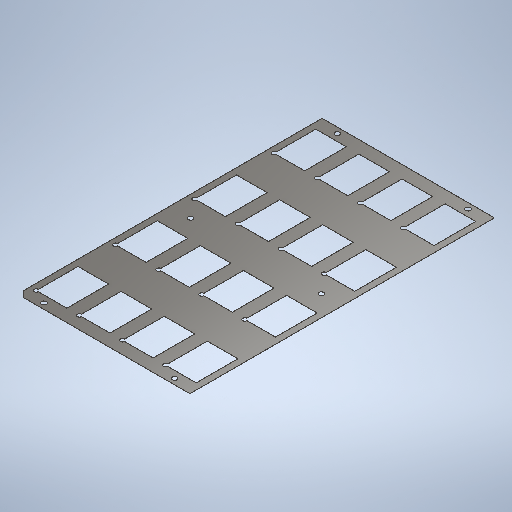
# Autodesk Inventor part: Assembly Stencil
Saved by Autodesk Inventor 2025 (Build 290162000, 162)
## iProperties
Created: 2021-01-11
Part Number: Assembly Stencil
Material: Stainless Steel
Document SubType Name: Modeling
Designer: caleb
Density: 8 g/cm^3
Appearance: Semi-Polished
Author: caleb
Autodesk Inventor part; units mm, degrees
ref_plane "YZ Plane" through (0, 0, 0) normal (1, 0, 0) x (0, 1, 0)
ref_plane "XZ Plane" through (0, 0, 0) normal (0, 1, 0) x (-1, 0, 0)
ref_plane "XY Plane" through (0, 0, 0) normal (0, 0, 1) x (1, 0, 0)
sketch "Sketch1" plane through (0, 0, 0) normal (0, 1, 0) x (-1, 0, 0)
  line L0 (-62, 109.5) -> (62, 109.5)
  line L1 (62, 109.5) -> (62, -109.5)
  line L2 (62, -109.5) -> (-62, -109.5)
  line L3 (-62, -109.5) -> (-62, 109.5)
  line L4 (-62, 109.5) -> (62, -109.5) construction
  line L5 (62, 109.5) -> (-62, -109.5) construction
  point P0 (0, 0)
  dimension "d0" = 219
  dimension "d1" = 124
  constraints: 12 end point, 2 midpoint, 2 parallel, 1 horizontal, 1 perpendicular
  measures "d0" distance of L0.end L1.end
  measures "d1" distance of L0.start L0.end
extrude "Extrusion1" add sketch "Sketch1" along normal blind 0.1
chamfer "Chamfer1" distance 4 angle 45 1 edges at (-62, 0.05, 109.5)
sketch "Sketch2" plane through (0, 0.1, 0) normal (0, 1, 0) x (1, 0, 0)
  line L0 (-35.5, -100.5) -> (-35.5, -70.5)
  line L1 (-35.5, -70.5) -> (-57.5, -70.5)
  line L2 (-62, 109.5) -> (-62, -109.5) projected
  line L3 (-62, -109.5) -> (62, -109.5) projected
  arc A0 (-57.5, -99) -> (-56, -100.5) centre (-57.5, -100.5) ccw
  line L4 (-35.5, -100.5) -> (-56, -100.5)
  line L5 (-57.5, -99) -> (-57.5, -70.5)
  line L6 (62, -109.5) -> (62, 109.5) projected
  line L7 (-35.5, -43.5) -> (-35.5, -13.5)
  line L8 (-35.5, -43.5) -> (-56, -43.5)
  line L9 (-35.5, -13.5) -> (-57.5, -13.5)
  line L10 (-57.5, -42) -> (-57.5, -13.5)
  arc A1 (-57.5, -42) -> (-56, -43.5) centre (-57.5, -43.5) ccw
  line L11 (-35.5, 13.5) -> (-35.5, 43.5)
  line L12 (-35.5, 13.5) -> (-56, 13.5)
  line L13 (-35.5, 43.5) -> (-57.5, 43.5)
  line L14 (-57.5, 15) -> (-57.5, 43.5)
  arc A2 (-57.5, 15) -> (-56, 13.5) centre (-57.5, 13.5) ccw
  line L15 (-35.5, 70.5) -> (-35.5, 100.5)
  line L16 (-35.5, 70.5) -> (-56, 70.5)
  line L17 (-35.5, 100.5) -> (-57.5, 100.5)
  line L18 (-57.5, 72) -> (-57.5, 100.5)
  arc A3 (-57.5, 72) -> (-56, 70.5) centre (-57.5, 70.5) ccw
  line L19 (-4.5, -100.5) -> (-4.5, -70.5)
  line L20 (-4.5, -100.5) -> (-25, -100.5)
  line L21 (-4.5, -70.5) -> (-26.5, -70.5)
  line L22 (-26.5, -99) -> (-26.5, -70.5)
  arc A4 (-26.5, -99) -> (-25, -100.5) centre (-26.5, -100.5) ccw
  line L23 (-4.5, -43.5) -> (-4.5, -13.5)
  line L24 (-4.5, -43.5) -> (-25, -43.5)
  line L25 (-4.5, -13.5) -> (-26.5, -13.5)
  line L26 (-26.5, -42) -> (-26.5, -13.5)
  arc A5 (-26.5, -42) -> (-25, -43.5) centre (-26.5, -43.5) ccw
  line L27 (-4.5, 13.5) -> (-4.5, 43.5)
  line L28 (-4.5, 13.5) -> (-25, 13.5)
  line L29 (-4.5, 43.5) -> (-26.5, 43.5)
  line L30 (-26.5, 15) -> (-26.5, 43.5)
  arc A6 (-26.5, 15) -> (-25, 13.5) centre (-26.5, 13.5) ccw
  line L31 (-4.5, 70.5) -> (-4.5, 100.5)
  line L32 (-4.5, 70.5) -> (-25, 70.5)
  line L33 (-4.5, 100.5) -> (-26.5, 100.5)
  line L34 (-26.5, 72) -> (-26.5, 100.5)
  arc A7 (-26.5, 72) -> (-25, 70.5) centre (-26.5, 70.5) ccw
  line L35 (26.5, -100.5) -> (26.5, -70.5)
  line L36 (26.5, -100.5) -> (6, -100.5)
  line L37 (26.5, -70.5) -> (4.5, -70.5)
  line L38 (4.5, -99) -> (4.5, -70.5)
  arc A8 (4.5, -99) -> (6, -100.5) centre (4.5, -100.5) ccw
  line L39 (26.5, -43.5) -> (26.5, -13.5)
  line L40 (26.5, -43.5) -> (6, -43.5)
  line L41 (26.5, -13.5) -> (4.5, -13.5)
  line L42 (4.5, -42) -> (4.5, -13.5)
  arc A9 (4.5, -42) -> (6, -43.5) centre (4.5, -43.5) ccw
  line L43 (26.5, 13.5) -> (26.5, 43.5)
  line L44 (26.5, 13.5) -> (6, 13.5)
  line L45 (26.5, 43.5) -> (4.5, 43.5)
  line L46 (4.5, 15) -> (4.5, 43.5)
  arc A10 (4.5, 15) -> (6, 13.5) centre (4.5, 13.5) ccw
  line L47 (26.5, 70.5) -> (26.5, 100.5)
  line L48 (26.5, 70.5) -> (6, 70.5)
  line L49 (26.5, 100.5) -> (4.5, 100.5)
  line L50 (4.5, 72) -> (4.5, 100.5)
  arc A11 (4.5, 72) -> (6, 70.5) centre (4.5, 70.5) ccw
  line L51 (57.5, -100.5) -> (57.5, -70.5)
  line L52 (57.5, -100.5) -> (37, -100.5)
  line L53 (57.5, -70.5) -> (35.5, -70.5)
  line L54 (35.5, -99) -> (35.5, -70.5)
  arc A12 (35.5, -99) -> (37, -100.5) centre (35.5, -100.5) ccw
  line L55 (57.5, -43.5) -> (57.5, -13.5)
  line L56 (57.5, -43.5) -> (37, -43.5)
  line L57 (57.5, -13.5) -> (35.5, -13.5)
  line L58 (35.5, -42) -> (35.5, -13.5)
  arc A13 (35.5, -42) -> (37, -43.5) centre (35.5, -43.5) ccw
  line L59 (57.5, 13.5) -> (57.5, 43.5)
  line L60 (57.5, 13.5) -> (37, 13.5)
  line L61 (57.5, 43.5) -> (35.5, 43.5)
  line L62 (35.5, 15) -> (35.5, 43.5)
  arc A14 (35.5, 15) -> (37, 13.5) centre (35.5, 13.5) ccw
  line L63 (57.5, 70.5) -> (57.5, 100.5)
  line L64 (57.5, 70.5) -> (37, 70.5)
  line L65 (57.5, 100.5) -> (35.5, 100.5)
  line L66 (35.5, 72) -> (35.5, 100.5)
  arc A15 (35.5, 72) -> (37, 70.5) centre (35.5, 70.5) ccw
  dimension "d46" = 1.5
  dimension "d47" = 30
  dimension "d50" = 9
  dimension "d51" = 4.5
  dimension "d62" = 57
  dimension "d65" = 31
  dimension "d77" = 22
  constraints: 128 end point, 32 point on circle, 16 centre point, 2 collinear, 2 horizontal, 2 vertical, 1 horizontal alignment, 1 perpendicular, 1 vertical alignment, 163 other
  measures "d46" radius of A0
  measures "d47" distance of L1.end A0.centre
  measures "d50" distance between parallel lines of L3 L4
  measures "d51" distance between parallel lines of L2 L5
  measures "d62" distance of L0.end L7.end
  measures "d65" distance of L0.end L19.end
  measures "d77" distance between parallel lines of L0 L5
extrude "Extrusion2" cut sketch "Sketch2" against normal through all
fillet "Fillet1" radius 1 5 edges at (62, 0.05, 109.5) (-58, 0.05, 109.5) (-62, 0.05, 105.5) (62, 0.05, -109.5) (-62, 0.05, -109.5)
sketch "Sketch3" plane through (0, 0.1, 0) normal (0, 1, 0) x (1, 0, 0)
  line L0 (-62, 108.5) -> (-62, -105.0858) projected
  line L1 (62, -108.5) -> (62, 108.5) projected
  line L2 (-57.5858, -109.5) -> (61, -109.5) projected
  line L3 (61, 109.5) -> (-61, 109.5) projected
  point P0 (0, 0)
  point P1 (-47, -105.5)
  point P2 (47, -105.5)
  point P3 (47, 105.5)
  point P4 (-47, 105.5)
  point P5 (-47, 0)
  point P6 (47, 0)
  dimension "d90" = 15
  dimension "d91" = 15
  dimension "d92" = 4
  dimension "d93" = 4
  constraints: 4 horizontal alignment, 4 vertical alignment
  measures "d90" distance from line of L0 point (-47, -105.5)
  measures "d91" distance from line of L1 point (47, -105.5)
  measures "d92" distance from line of L2 point (-47, -105.5)
  measures "d93" distance from line of L3 point (-47, 105.5)
hole "Hole1" at (-47, 0.1, 105.5) at (47, 0.1, 105.5) at (47, 0.1, -105.5) at (-47, 0.1, -105.5) at (-47, 0.1, 0) at (47, 0.1, 0) direction (0, -1, 0) diameter 3.4 end through all clearance for "Flat Head Machine Screw" size "M3" standard "Ansi Metric M Profile"
body "Solid1"
